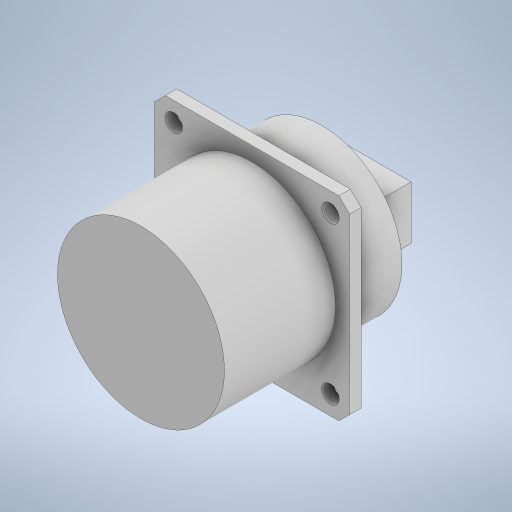
# Autodesk Inventor part: RJFTV21 X Amphenol Connector
Saved by Autodesk Inventor 2023 (Build 270158000, 158)
## iProperties
Created: 2023-05-22
Part Number: RJFTV21 X Amphenol Connector
Material: Generic
Document SubType Name: Modeling
Designer: Louis
Density: 1 g/cm^3
Appearance: Default
Author: Louis
Autodesk Inventor part; units mm, degrees
ref_plane "YZ Plane" through (0, 0, 0) normal (1, 0, 0) x (0, 1, 0)
ref_plane "XZ Plane" through (0, 0, 0) normal (0, 1, 0) x (-1, 0, 0)
ref_plane "XY Plane" through (0, 0, 0) normal (0, 0, 1) x (1, 0, 0)
sketch "Sketch1" plane through (0, 0, 0) normal (0, 0, 1) x (1, 0, 0)
  line L0 (-18.265, 18.265) -> (18.265, 18.265)
  line L1 (18.265, 18.265) -> (18.265, -18.265)
  line L2 (18.265, -18.265) -> (-18.265, -18.265)
  line L3 (-18.265, -18.265) -> (-18.265, 18.265)
  point P0 (0, 0)
  point P1 (0, 18.265)
  point P2 (-18.265, 0)
  dimension "d0" = 36.53
  dimension "d1" = 36.53
  constraints: 8 end point, 2 midpoint, 2 parallel, 1 horizontal, 1 horizontal alignment, 1 perpendicular, 1 vertical alignment
  measures "d0" distance of L0.start L0.end
  measures "d1" distance of L0.end L1.end
extrude "Extrusion1" add sketch "Sketch1" along normal blind 2.16
chamfer "Chamfer1" distance 2 angle 45 4 edges at (18.265, 18.265, 1.08) (-18.265, 18.265, 1.08) (-18.265, -18.265, 1.08) (18.265, -18.265, 1.08)
sketch "Sketch2" plane through (0, 0, 2.16) normal (0, 0, 1) x (1, 0, 0)
  line L0 (-14.68, 14.68) -> (14.68, 14.68)
  line L1 (14.68, 14.68) -> (14.68, -14.68)
  line L2 (14.68, -14.68) -> (-14.68, -14.68)
  line L3 (-14.68, -14.68) -> (-14.68, 14.68)
  point P0 (0, 0)
  point P1 (0, 14.68)
  point P2 (-14.68, 0)
  dimension "d7" = 29.36
  constraints: 8 end point, 4 coincident, 2 midpoint, 2 parallel, 2 perpendicular, 1 horizontal, 1 horizontal alignment, 1 vertical alignment
  measures "d7" distance of L0.start L0.end
hole "Hole1" at (-14.68, 14.68, 2.16) at (14.68, 14.68, 2.16) at (-14.68, -14.68, 2.16) at (14.68, -14.68, 2.16) direction (0, 0, -1) diameter 3.25 end through all
sketch "Sketch3" plane through (0, 0, 2.16) normal (0, 0, 1) x (1, 0, 0)
  circle A0 centre (0, 0) radius 15.625
  dimension "d15" = 31.25
  constraints: 1 centre point, 1 coincident
  measures "d15" diameter of A0
extrude "Extrusion2" add sketch "Sketch3" along normal blind 20.83
sketch "Sketch4" plane through (0, 0, 0) normal (0, 0, -1) x (-1, 0, 0)
  circle A0 centre (0, 0) radius 15
  dimension "d18" = 30
  constraints: 1 centre point, 1 coincident
  measures "d18" diameter of A0
extrude "Extrusion3" add sketch "Sketch4" along normal blind 10.9
sketch "Sketch5" plane through (0, 0, -10.9) normal (0, 0, -1) x (-1, 0, 0)
  line L0 (-7.5, 5) -> (7.5, 5)
  line L1 (7.5, 5) -> (7.5, -5)
  line L2 (7.5, -5) -> (-7.5, -5)
  line L3 (-7.5, -5) -> (-7.5, 5)
  point P0 (0, 0)
  point P1 (0, 5)
  point P2 (7.5, 0)
  dimension "d21" = 15
  dimension "d22" = 10
  constraints: 8 end point, 2 midpoint, 2 parallel, 1 horizontal, 1 horizontal alignment, 1 perpendicular, 1 vertical alignment
  measures "d21" distance of L0.start L0.end
  measures "d22" distance of L0.end L1.end
extrude "Extrusion4" add sketch "Sketch5" along normal blind 9.21
body "Solid1"
